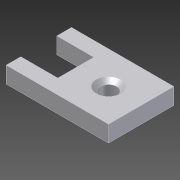
# Autodesk Inventor part: Gabel02
Saved by Autodesk Inventor 2013 (Build 170138000, 138)
## iProperties
Created: 2006-09-13
Part Number: Gabel02
Document SubType Name: Modeling
Designer: acad
Manufacturer: Standard
Standards Organization: Custom
Material: Allgemein
Density: 1 g/cm^3
Author: acad
Autodesk Inventor part; units mm, degrees
ref_plane "YZ Plane" through (0, 0, 0) normal (1, 0, 0) x (0, 1, 0)
ref_plane "XZ Plane" through (0, 0, 0) normal (0, 1, 0) x (-1, 0, 0)
ref_plane "XY Plane" through (0, 0, 0) normal (0, 0, 1) x (1, 0, 0)
sketch "Skizze1" plane through (0, 0, 0) normal (0, 0, 1) x (1, 0, 0)
  line L0 (13.6139, 4) -> (13.6139, 0) projected
  line L1 (13.6139, 0) -> (30.3639, 0) projected
  line L2 (30.3639, 0) -> (30.3639, 4) projected
  line L3 (13.6139, 4) -> (30.3639, 4) projected
  circle A0 centre (16.6139, 2) radius 1.6 projected
  circle A1 centre (16.6139, 2) radius 1.1 projected
  line L4 (21.7139, 0) -> (21.7139, 4)
  line L5 (15.452, 4) -> (15.452, 3.1)
  line L6 (15.452, 3.1) -> (17.7139, 3.1)
  line L7 (17.7139, 3.1) -> (17.7139, 0.9)
  line L8 (17.7139, 0.9) -> (15.452, 0.9)
  line L9 (15.452, 0.9) -> (15.452, 0)
  point P0 (19.7139, 2)
  dimension "d0" = 4
  dimension "d1" = 2
  dimension "d2" = 2
  dimension "d18" = 6.2619
  constraints: 12 end point, 4 point on line, 3 parallel, 3 perpendicular, 3 tangent, 2 point on circle
  measures "d0" distance between parallel lines of L7 L4
  measures "d1" distance from line of L3 point (19.714, 2)
  measures "d2" distance from line of L4 point (19.714, 2)
  measures "d18" distance between parallel lines of L4 L9
extrude "Extrusion1" add sketch "Skizze1" along normal blind 1 contours L3 L4 L1 L9 A0 L5 | A0 L8 L7 L6
sketch "Skizze3" plane through (0, 0, 1) normal (0, 0, 1) x (1, 0, 0)
  line L0 (21.7139, 4) -> (21.7139, 0) projected
  line L1 (15.452, 4) -> (21.7139, 4) projected
  point P0 (19.7139, 2)
  dimension "d7" = 2
  dimension "d8" = 2
  measures "d7" distance from line of point (19.714, 2) L0
  measures "d8" distance from line of L1 point (19.714, 2)
hole "Bohrung1" at (19.7139, 2, 1) direction (0, 0, -1) diameter 1 end through all countersink diameter 1.5 countersink angle 90
